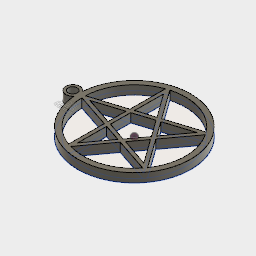
gj v1 (Autodesk Fusion 360 design; units mm, degrees)
Autodesk Fusion 360 part; units mm, degrees
sketch "草图1" plane through (0, 0, 0) normal (0, 1, 0) x (1, 0, 0)
  circle A0 centre (0, 0) radius 31.4721
  circle A1 centre (0, 0) radius 28.4721
  line L0 (-24.9993, 0.1898) -> (-9.7628, -4.889)
  line L1 (-7.7678, -5.554) -> (20.1133, -14.8477)
  line L2 (-28.4619, -0.7642) -> (-9.7788, -6.9919)
  line L3 (-7.7838, -7.6569) -> (22.311, -17.6885)
  line L4 (20.3364, 14.5407) -> (2.8818, -9.1039)
  line L5 (1.6329, -10.7958) -> (-7.9057, -23.7171)
  line L6 (23.7172, 15.753) -> (4.8768, -9.7689)
  line L7 (3.6279, -11.4608) -> (-8.0684, -27.305)
  line L8 (-7.6529, 27.4244) -> (10.7978, 1.6194)
  line L9 (12.0209, -0.0913) -> (23.4753, -16.1112)
  line L10 (-7.5447, 23.8344) -> (9.5489, -0.0725)
  line L11 (10.772, -1.7831) -> (20.1133, -14.8477)
  line L12 (-24.9993, 0.1898) -> (3.0197, 9.0591)
  line L13 (5.0246, 9.6938) -> (20.3364, 14.5407)
  line L14 (-28.447, 1.1962) -> (1.7966, 10.7698)
  line L15 (3.8015, 11.4044) -> (22.577, 17.3477)
  line L16 (-9.522, 26.8327) -> (-9.6715, 7.1396)
  line L17 (-9.6875, 5.0367) -> (-9.9283, -26.685)
  line L18 (-7.5447, 23.8344) -> (-7.6666, 7.7742)
  line L19 (-7.6826, 5.6713) -> (-7.9057, -23.7171)
extrude "拉伸1" add sketch "草图1" along normal blind 5 contours A1 L0 L2 L10 L12 L14 L17 makes body 1
extrude "拉伸2" add sketch "草图1" along normal blind 5 bodies 1
extrude "拉伸3" add sketch "草图1" along normal blind 5 contours A1 L1 L3 L6 L9 L11 L19 bodies 1
extrude "拉伸4" add sketch "草图1" along normal blind 5 contours A1 L3 L5 L7 L12 L17 L19 bodies 1
extrude "拉伸5" add sketch "草图1" along normal blind 5 contours A1 L1 L4 L6 L8 L13 L15 bodies 1
extrude "拉伸6" add sketch "草图1" along normal blind 5 contours A1 L4 L8 L10 L14 L16 L18 bodies 1
sketch "草图2" plane through (0, 0, 0) normal (0, 1, 0) x (1, 0, 0)
  circle A0 centre (-80, 5) radius 4
  circle A1 centre (-80, 5) radius 2.5
extrude "拉伸7" add sketch "草图2" along normal blind 5 separate body makes body 2
move_body "移动1" bodies 2 to x (1, 0, 0) y (0, 1, 0) z (0, 0, 1) at (45.4441, 0, 4.7092)
combine "合并1" operation add target body 2 tool bodies 1
